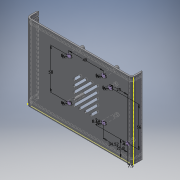
# Autodesk Inventor part: case-bottom
Saved by Autodesk Inventor 2017 (Build 210142000, 142)
## iProperties
Created: 2020-10-01
Part Number: case-bottom
Material: Generic
Document SubType Name: Modeling
Designer: jferner
Density: 1 g/cm^3
Appearance: Default
caseBottomDepth: 108.000 mm
caseBottomHeight: 16.000 mm
caseBottomWidth: 150.000 mm
thickness: 2.000 mm
fillet: 5.000 mm
frontBackOffset: -5.000 mm
filletInner: 3.000 mm
filletMid: 4.000 mm
lipHeight: 1.000 mm
Author: jferner
Autodesk Inventor part; units mm, degrees
ref_plane "YZ Plane" through (0, 0, 0) normal (1, 0, 0) x (0, 1, 0)
ref_plane "XZ Plane" through (0, 0, 0) normal (0, 1, 0) x (-1, 0, 0)
ref_plane "XY Plane" through (0, 0, 0) normal (0, 0, 1) x (1, 0, 0)
sketch "Sketch1" plane through (0, 0, 0) normal (0, 0, 1) x (1, 0, 0)
  line L0 (0, 16) -> (0, 5)
  line L1 (5, 0) -> (145, 0)
  line L2 (150, 5) -> (150, 16)
  arc A0 (0, 5) -> (5, 0) centre (5, 5) ccw
  arc A1 (145, 0) -> (150, 5) centre (145, 5) ccw
  line L3 (2, 16) -> (2, 5)
  arc A2 (2, 5) -> (5, 2) centre (5, 5) ccw
  line L4 (5, 2) -> (145, 2)
  arc A3 (145, 2) -> (148, 5) centre (145, 5) ccw
  line L5 (148, 5) -> (148, 16)
  line L6 (0, 16) -> (2, 16)
  line L7 (148, 16) -> (150, 16)
  point P0 (0, 0)
  dimension "fillet" = 5
  dimension "thickness" = 2
  dimension "caseBottomWidth" = 150
  dimension "caseBottomHeight" = 16
  constraints: 16 end point, 8 point on circle, 4 centre point, 4 perpendicular, 4 tangent, 2 collinear, 2 point on line, 1 equal radius, 1 horizontal, 1 vertical, 4 other
  measures "fillet" radius of A0
  measures "thickness" distance between parallel lines of L0 L3
  measures "caseBottomWidth" distance between parallel lines of L2 L0
  measures "caseBottomHeight" distance between parallel lines of L6 L1
extrude "Extrusion1" add sketch "Sketch1" along normal blind 108
ref_plane "Work Plane1" through (0, 0, 103) normal (0, 0, 1) x (1, 0, 0)
sketch "Sketch3" plane through (0, 0, 103) normal (0, 0, 1) x (1, 0, 0)
  line L0 (2, 16) -> (1, 16)
  line L1 (2, 16) -> (2, 5)
  line L2 (1, 16) -> (1, 5)
  line L3 (145, 2) -> (5, 2) projected
  line L4 (145, 2) -> (5, 2)
  line L5 (148, 16) -> (148, 5) projected
  line L6 (148, 16) -> (148, 5)
  line L7 (148, 16) -> (149, 16)
  line L8 (149, 16) -> (149, 5)
  line L9 (5, 1) -> (145, 1)
  arc A0 (2, 5) -> (5, 2) centre (5, 5) ccw
  arc A1 (145, 2) -> (148, 5) centre (145, 5) ccw
  arc A2 (1, 5) -> (5, 1) centre (5, 5) ccw
  arc A3 (145, 1) -> (149, 5) centre (145, 5) ccw
  point P0 (0, 0)
  dimension "d8" = 1
  dimension "d9" = 1
  dimension "d10" = 1
  dimension "filletInner" = 3
  dimension "filletMid" = 4
  constraints: 16 end point, 8 point on circle, 8 tangent, 4 centre point, 4 horizontal, 3 vertical, 2 equal radius, 1 collinear, 1 parallel
  measures "d8" distance of L0.start L0.end
  measures "d9" distance of L5.start L7.end
  measures "d10" distance between parallel lines of L9 L4
  measures "filletInner" radius of A0
  measures "filletMid" radius of A2
extrude "Extrusion2" cut sketch "Sketch3" against normal blind 2
ref_plane "Work Plane2" through (0, 0, 5) normal (0, 0, -1) x (-1, 0, 0)
sketch "Sketch5" plane through (0, 0, 5) normal (0, 0, -1) x (-1, 0, 0)
  line L0 (-150, 16) -> (-148, 16) projected
  line L1 (-148, 16) -> (-148, 5)
  line L2 (-149, 16) -> (-149, 5)
  line L3 (-2, 5) -> (-2, 16) projected
  line L4 (-2, 16) -> (-2, 5)
  line L5 (-2, 16) -> (0, 16) projected
  line L6 (-1, 16) -> (-1, 5)
  line L7 (-145, 2) -> (-5, 2)
  line L8 (-145, 1) -> (-5, 1)
  line L9 (-145, 2) -> (-5, 2) projected
  arc A0 (-148, 5) -> (-145, 2) centre (-145, 5) ccw
  arc A1 (-5, 2) -> (-2, 5) centre (-5, 5) ccw
  arc A2 (-149, 5) -> (-145, 1) centre (-145, 5) ccw
  arc A3 (-5, 1) -> (-1, 5) centre (-5, 5) ccw
  point P0 (0, 0)
  dimension "d21" = 1
  dimension "d22" = 3
  dimension "d23" = 4
  constraints: 12 end point, 8 point on circle, 8 tangent, 4 centre point, 4 vertical, 2 equal radius, 2 horizontal, 2 midpoint, 1 collinear
  measures "d21" distance between parallel lines of L7 L8
  measures "d22" radius of A0
  measures "d23" radius of A2
extrude "Extrusion4" cut sketch "Sketch5" against normal blind 2
sketch "Sketch6" plane through (0, 0, 0) normal (0, 0, -1) x (-1, 0, 0)
  line L0 (-149, 16) -> (-149, 5) projected
  line L1 (-150, 5) -> (-150, 16) projected
  line L2 (-149, 16) -> (-150, 16)
  line L3 (-150, 16) -> (-150, 15)
  line L4 (-150, 15) -> (-149, 15)
  line L5 (-149, 15) -> (-149, 16)
  line L6 (-1, 16) -> (-1, 5) projected
  line L7 (0, 16) -> (-1, 16)
  line L8 (-1, 16) -> (-1, 15)
  line L9 (-1, 15) -> (0, 15)
  line L10 (0, 15) -> (0, 16)
  line L11 (0, 16) -> (0, 5) projected
  line L12 (-2, 16) -> (0, 16) projected
  point P0 (0, 0)
  dimension "lipHeight" = 1
  constraints: 16 end point, 4 parallel, 3 collinear, 2 horizontal, 2 perpendicular, 2 point on line
  measures "lipHeight" distance between parallel lines of L2 L4
extrude "Extrusion5" cut sketch "Sketch6" against normal through all
sketch "Sketch7" plane through (5, 2, 0) normal (0, 1, 0) x (1, 0, 0)
  circle A0 centre (137.1, -22.8) radius 2.25
  circle A1 centre (137.1, -22.8) radius 1.25
  circle A2 centre (102.58, -30.94) radius 2.25
  circle A3 centre (102.58, -30.94) radius 1.25
  circle A4 centre (102.58, -88.94) radius 2.25
  circle A5 centre (102.58, -88.94) radius 1.25
  circle A6 centre (53.58, -88.94) radius 2.25
  circle A7 centre (53.58, -88.94) radius 1.25
  circle A8 centre (53.58, -30.94) radius 2.25
  circle A9 centre (53.58, -30.94) radius 1.25
  circle A10 centre (112.1, -78.8) radius 2.25
  circle A11 centre (112.1, -78.8) radius 1.25
  line L0 (140, 0) -> (0, 0) projected
  line L1 (145, 0) -> (145, -108) projected
  point P0 (-5, 0)
  dimension "holeSupportDiameter" = 4.5
  dimension "holeDiameter" = 2.5
  dimension "d31" = 4.5
  dimension "d32" = 2.5
  dimension "d33" = 4.5
  dimension "d34" = 2.5
  dimension "d35" = 4.5
  dimension "d36" = 2.5
  dimension "d37" = 4.5
  dimension "d38" = 2.5
  dimension "d39" = 58
  dimension "d40" = 49
  dimension "d43" = 4.5
  dimension "d44" = 2.5
  dimension "d45" = 25
  dimension "d46" = 56
  dimension "d59" = 22.8
  dimension "d60" = 7.9
  dimension "d61" = 34.52
  dimension "d62" = 8.14
  constraints: 12 centre point, 6 coincident, 2 horizontal alignment, 2 vertical alignment
  measures "holeSupportDiameter" diameter of A0
  measures "holeDiameter" diameter of A1
  measures "d31" diameter of A2
  measures "d32" diameter of A3
  measures "d33" diameter of A4
  measures "d34" diameter of A5
  measures "d35" diameter of A6
  measures "d36" diameter of A7
  measures "d37" diameter of A8
  measures "d38" diameter of A9
  measures "d39" distance of A6.centre A8.centre
  measures "d40" distance of A6.centre A4.centre
  measures "d43" diameter of A10
  measures "d44" diameter of A11
  measures "d45" horizontal distance of A10.centre A0.centre
  measures "d46" vertical distance of A10.centre A0.centre
  measures "d59" distance from line of L0 A0.centre
  measures "d60" distance from line of L1 A0.centre
  measures "d61" horizontal distance of A0.centre A2.centre
  measures "d62" vertical distance of A2.centre A0.centre
extrude "Extrusion6" add sketch "Sketch7" along normal blind 20.5 contours A2 | A3 | A4 | A5 | A6 | A7 | A8 | A9
extrude "Extrusion7" add sketch "Sketch7" along normal blind 9.4 contours A0 | A1 | A10 | A11
sketch "Sketch8" plane through (142.1, 11.4, 22.8) normal (0, 1, 0) x (1, 0, 0)
  circle A0 centre (0, 0) radius 2.25 projected
  circle A1 centre (0, 0) radius 1.25
  circle A2 centre (-25, -56) radius 1.25
  circle A3 centre (-25, -56) radius 2.25 projected
  circle A4 centre (0, 0) radius 2.25 projected
  point P0 (-142.1, 22.8)
  point P1 (2.2499, -0.0186)
  point P2 (2.2499, 0.0186)
  dimension "d49" = 2.5
  dimension "d50" = 2.5
  constraints: 2 centre point, 2 concentric, 1 coincident
  measures "d49" diameter of A1
  measures "d50" diameter of A2
extrude "Extrusion8" cut sketch "Sketch8" against normal blind 5 contours A1 | A2
sketch "Sketch9" plane through (107.58, 22.5, 30.94) normal (0, 1, 0) x (1, 0, 0)
  circle A0 centre (0, -58) radius 1.25
  circle A1 centre (0, 0) radius 1.25
  circle A2 centre (-49, 0) radius 1.25
  circle A3 centre (-49, -58) radius 2.25 projected
  circle A4 centre (-49, -58) radius 1.25
  circle A5 centre (0, -58) radius 2.25 projected
  circle A6 centre (0, 0) radius 2.25 projected
  circle A7 centre (-49, 0) radius 2.25 projected
  point P0 (-107.58, 30.94)
  dimension "d53" = 2.5
  dimension "d54" = 2.5
  dimension "d55" = 2.5
  dimension "d56" = 2.5
  constraints: 4 centre point, 3 concentric, 1 coincident
  measures "d53" diameter of A0
  measures "d54" diameter of A4
  measures "d55" diameter of A1
  measures "d56" diameter of A2
extrude "Extrusion9" cut sketch "Sketch9" against normal blind 5 contours A0 | A1 | A2 | A4
sketch "Sketch11" plane through (5, 0, 0) normal (0, -1, 0) x (1, 0, 0)
  line L0 (145, 0) -> (145, 108) projected
  line L1 (0, 108) -> (140, 108) projected
  line L2 (88.0854, 31.9636) -> (96.038, 39.9162)
  line L3 (85.9338, 34.0551) -> (93.9393, 42.0607)
  line L4 (96.1987, 48.0774) -> (80.0607, 31.9393)
  line L5 (77.9393, 34.0607) -> (93.9393, 50.0607)
  line L6 (72.0607, 31.9393) -> (96.0607, 55.9393)
  line L7 (93.9393, 58.0607) -> (69.9393, 34.0607)
  line L8 (64.0607, 31.9393) -> (96.0607, 63.9393)
  line L9 (93.9393, 66.0607) -> (61.9393, 34.0607)
  line L10 (64.0607, 39.9393) -> (96.0607, 71.9393)
  line L11 (93.9393, 74.0607) -> (61.9393, 42.0607)
  line L12 (64.0607, 47.9393) -> (88.0607, 71.9393)
  line L13 (85.9393, 74.0607) -> (61.9393, 50.0607)
  line L14 (64.0607, 55.9393) -> (80.0607, 71.9393)
  line L15 (77.9393, 74.0607) -> (61.9393, 58.0607)
  line L16 (64.0607, 63.9393) -> (72.0607, 71.9393)
  line L17 (69.9393, 74.0607) -> (61.9393, 66.0607)
  arc A0 (85.9338, 34.0551) -> (88.0854, 31.9636) centre (87.0244, 33.0246) ccw
  arc A1 (96.038, 39.9162) -> (93.9393, 42.0607) centre (94.9771, 40.9771) ccw
  arc A2 (96.1987, 48.0774) -> (93.9393, 50.0607) centre (95.1336, 49.1426) ccw
  arc A3 (96.0607, 55.9393) -> (93.9393, 58.0607) centre (95, 57) ccw
  arc A4 (96.0607, 63.9393) -> (93.9393, 66.0607) centre (95, 65) ccw
  arc A5 (96.0607, 71.9393) -> (93.9393, 74.0607) centre (95, 73) ccw
  arc A6 (88.0607, 71.9393) -> (85.9393, 74.0607) centre (87, 73) ccw
  arc A7 (80.0607, 71.9393) -> (77.9393, 74.0607) centre (79, 73) ccw
  arc A8 (72.0607, 71.9393) -> (69.9393, 74.0607) centre (71, 73) ccw
  arc A9 (61.9393, 66.0607) -> (64.0607, 63.9393) centre (63, 65) ccw
  arc A10 (61.9393, 58.0607) -> (64.0607, 55.9393) centre (63, 57) ccw
  arc A11 (61.9393, 50.0607) -> (64.0607, 47.9393) centre (63, 49) ccw
  arc A12 (61.9393, 42.0607) -> (64.0607, 39.9393) centre (63, 41) ccw
  arc A13 (61.9393, 34.0607) -> (64.0607, 31.9393) centre (63, 33) ccw
  arc A14 (69.9393, 34.0607) -> (72.0607, 31.9393) centre (71, 33) ccw
  arc A15 (77.9393, 34.0607) -> (80.0607, 31.9393) centre (79, 33) ccw
  point P0 (-5, 0)
  constraints: 32 end point, 32 point on circle, 29 tangent, 16 centre point, 1 parallel
extrude "Extrusion11" cut sketch "Sketch11" against normal blind 4
equation "\"d8\" = 0.5 * thickness"
equation "\"d9\" = 0.5 * thickness"
equation "\"d10\" = 0.5 * thickness"
equation "\"d13\" = thickness"
equation "\"d21\" = 0.5 * thickness"
equation "\"d22\" = filletInner"
equation "\"d23\" = filletMid"
equation "\"d24\" = thickness"
equation "\"d31\" = holeSupportDiameter"
equation "\"d32\" = holeDiameter"
equation "\"d33\" = holeSupportDiameter"
equation "\"d34\" = holeDiameter"
equation "\"d35\" = holeSupportDiameter"
equation "\"d36\" = holeDiameter"
equation "\"d37\" = holeSupportDiameter"
equation "\"d38\" = holeDiameter"
equation "\"d43\" = holeSupportDiameter"
equation "\"d44\" = holeDiameter"
equation "\"d49\" = holeDiameter"
equation "\"d50\" = holeDiameter"
equation "\"d53\" = holeDiameter"
equation "\"d54\" = holeDiameter"
equation "\"d55\" = holeDiameter"
equation "\"d56\" = holeDiameter"
equation "\"d57\" = holeDepth"
equation "\"d139\" = 2 * thickness"
equation "\"d15\" = frontBackOffset"
equation "\"holeDepth\" = 5"
equation "\"frontBackOffset\" = -5"
body "Solid1"
